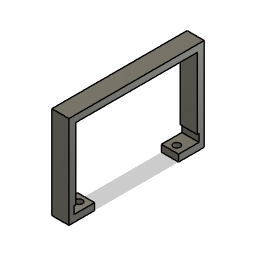
support_etage v3 (Autodesk Fusion 360 design; units mm, degrees)
Autodesk Fusion 360 part; units mm, degrees
sketch "Sketch1" plane through (0, 0, 0) normal (1, 0, 0) x (0, 0, -1)
  line L0 (0, 0) -> (15, 0)
  line L1 (15, 0) -> (15, 4)
  line L2 (15, 4) -> (3, 4)
  line L3 (3, 4) -> (3, 8.4)
  line L4 (3, 8.4) -> (4, 8.4)
  line L5 (4, 8.4) -> (4, 50)
  line L6 (4, 50) -> (39.5, 50)
  line L7 (39.5, 54) -> (0, 54)
  line L8 (0, 54) -> (0, 0)
  line L9 (39.5, 54) -> (39.5, 50) construction
  line L10 (64, 0) -> (64, 4)
  line L11 (79, 0) -> (64, 0)
  line L12 (75, 8.4) -> (75, 50)
  line L13 (76, 4) -> (76, 8.4)
  line L14 (76, 8.4) -> (75, 8.4)
  line L15 (79, 54) -> (79, 0)
  line L16 (64, 4) -> (76, 4)
  line L17 (75, 50) -> (39.5, 50)
  line L18 (39.5, 54) -> (79, 54)
  point P0 (79, 0)
  dimension "d1" = 4.4
  dimension "d3" = 4
  dimension "d4" = 4
  dimension "d5" = 50
  dimension "d7" = 73
  dimension "d8" = 4
  dimension "d11" = 3
  dimension "d12" = 15
  constraint coincident L0.start L8.end
  constraint horizontal L0
  constraint perpendicular L0 L1
  constraint perpendicular L1 L2
  constraint vertical L3
  constraint perpendicular L3 L4
  constraint perpendicular L4 L5
  constraint perpendicular L0 L8
  constraint horizontal L7
  constraint horizontal L6
  constraint vertical L9
  constraint symmetric L0.start L9 L11.start
  constraint symmetric L0.start L9 P0
  constraint symmetric L0.end L9 L10.start
  constraint symmetric L1.end L9 L10.end
  constraint symmetric L2.end L9 L13.start
  constraint symmetric L3.end L9 L13.end
  constraint symmetric L4.end L9 L12.start
  constraint symmetric L5.end L9 L12.end
  constraint symmetric L6.end L9 L17.end
  constraint symmetric L7.start L9 L18.start
  constraint symmetric L7.end L9 L15.start
  measures "d1" distance of L2 L4
  measures "d3" distance of L5 L8
  measures "d4" distance of L6 L7
  measures "d5" distance of L0 L6
  measures "d7" distance of L3 L13
  measures "d8" distance of L0 L2
  measures "d11" distance of L3 L8
  measures "d12" distance of L1 L8
extrude "Extrude1" add sketch "Sketch1" along normal blind 10
sketch "Sketch2" plane through (0, 0, 0) normal (0, -1, 0) x (1, 0, 0)
  line L0 (0, 0) -> (0, -15)
  line L1 (0, -15) -> (10, -15)
  line L2 (10, -15) -> (10, 0)
  line L3 (10, 0) -> (0, 0)
  circle A0 centre (5, -11) radius 2
  line L4 (5, -15) -> (5, 0) construction
  dimension "d15" = 4
  dimension "d18" = 11
  constraint midpoint L1 L4.start
  constraint midpoint L3 L4.end
  constraint coincident A0.centre L4
  measures "d15" diameter of A0
  measures "d18" distance of L3 A0.centre
extrude "Extrude2" cut sketch "Sketch2" against normal up to surface (4 mm away) contours A0
ref_plane "WorkPlane1" through (5, 27, -39.5) normal (0, 0, -1) x (0, 1, 0)
mirror "Mirror1" about plane through (5, 27, -39.5) normal (0, 0, -1) of "Extrude2"
